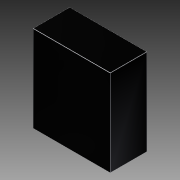
# Autodesk Inventor part: controller
Saved by Autodesk Inventor 2015 (Build 190159000, 159)
## iProperties
Created: 2015-12-24
Part Number: controller
Material: ABS プラスチック
Document SubType Name: Modeling
Designer: Ryo
Density: 1.06 g/cm^3
Appearance: 滑らか - 白
Author: Ryo
Autodesk Inventor part; units mm, degrees
ref_plane "YZ Plane" through (0, 0, 0) normal (1, 0, 0) x (0, 1, 0)
ref_plane "XZ Plane" through (0, 0, 0) normal (0, 1, 0) x (-1, 0, 0)
ref_plane "XY Plane" through (0, 0, 0) normal (0, 0, 1) x (1, 0, 0)
sketch "スケッチ1" plane through (0, 0, 0) normal (0, 1, 0) x (-1, 0, 0)
  line L0 (-210, 235) -> (210, 235)
  line L1 (210, 235) -> (210, -235)
  line L2 (210, -235) -> (-210, -235)
  line L3 (-210, -235) -> (-210, 235)
  line L4 (-210, 235) -> (210, -235) construction
  line L5 (210, 235) -> (-210, -235) construction
  point P0 (0, 0)
  dimension "d0" = 420
  dimension "d1" = 470
  constraints: 12 end point, 2 midpoint, 2 parallel, 1 horizontal, 1 perpendicular
  measures "d0" distance of L1.end L2.end
  measures "d1" distance between parallel lines of L2 L0
extrude "押し出し1" add sketch "スケッチ1" along normal blind 200
fillet "フィレット1" radius 2 12 edges at (-210, 100, 235) (210, 100, 235) (210, 200, 0) (0, 200, 235) (0, 0, 235) (210, 0, 0) (210, 100, -235) (0, 200, -235) (-210, 200, 0) (-210, 100, -235) (-210, 0, 0) (0, 0, -235)
